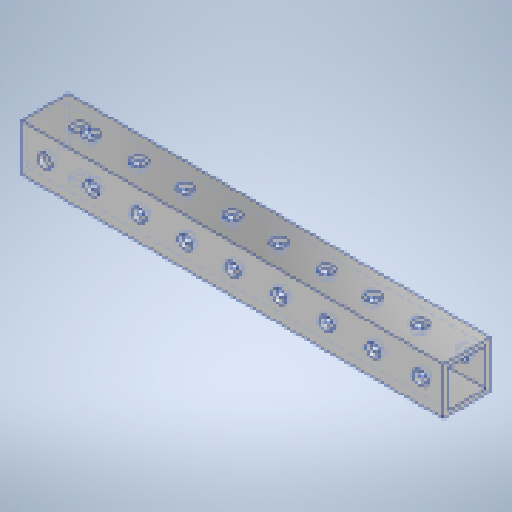
# Autodesk Inventor part: 10x10x60
Saved by Autodesk Inventor 2025 (Build 290162000, 162)
## iProperties
Created: 2025-03-04
Part Number: 10x10x60
Material: アルミニウム 6061
Document SubType Name: Modeling
Designer: Zhopa
Density: 2.7 g/cm^3
Appearance: アルミニウム - フラット
Mass: 8.06397 g
Surface Area: 63.7758 cm^2
Volume: 2.98666 cm^3
Author: Zhopa
Autodesk Inventor part; units mm, degrees
ref_plane "YZ Plane" through (0, 0, 0) normal (1, 0, 0) x (0, 1, 0)
ref_plane "XZ Plane" through (0, 0, 0) normal (0, 1, 0) x (-1, 0, 0)
ref_plane "XY Plane" through (0, 0, 0) normal (0, 0, 1) x (1, 0, 0)
sketch "Sketch1" plane through (0, 0, 0) normal (1, 0, 0) x (0, 1, 0)
  line L0 (-5, -5) -> (5, -5)
  line L1 (5, -5) -> (5, 5)
  line L2 (5, 5) -> (-5, 5)
  line L3 (-5, 5) -> (-5, -5)
  line L4 (-5, -5) -> (5, 5) construction
  line L5 (5, -5) -> (-5, 5) construction
  line L6 (-4, -4) -> (4, -4)
  line L7 (4, -4) -> (4, 4)
  line L8 (4, 4) -> (-4, 4)
  line L9 (-4, 4) -> (-4, -4)
  line L10 (-4, -4) -> (4, 4) construction
  line L11 (4, -4) -> (-4, 4) construction
  point P0 (0, 0)
  dimension "d0" = 10
  dimension "d1" = 10
  dimension "d2" = 8
  dimension "d3" = 8
  constraints: 24 end point, 4 midpoint, 4 parallel, 2 horizontal, 2 perpendicular
  measures "d0" distance of L2.end L1.end
  measures "d1" distance of L1.end L0.end
  measures "d2" distance of L8.end L7.end
  measures "d3" distance of L7.end L6.end
extrude "Extrusion1" add sketch "Sketch1" along normal blind 90
sketch "Sketch2" plane through (0, -5, 5) normal (0, 0, 1) x (1, 0, 0)
  line L0 (90, 10) -> (90, 0) projected
  line L1 (0, 10) -> (0, 0) projected
  line L2 (5, 5) -> (25.8215, 5)
  point P0 (0, 5)
  point P1 (15, 5)
  point P2 (15, 5)
  point P3 (25, 5)
  point P4 (25, 5)
  point P5 (35, 5)
  point P6 (35, 5)
  point P7 (45, 5)
  point P8 (45, 5)
  point P9 (55, 5)
  point P10 (55, 5)
  point P11 (65, 5)
  point P12 (65, 5)
  point P13 (75, 5)
  point P14 (75, 5)
  point P15 (85, 5)
  dimension "d7" = 5
  dimension "d15" = 10
  dimension "d18" = 10
  constraints: 2 end point, 2 horizontal, 14 other
  measures "d7" distance from line of L1 L2.start
  measures "d15" distance of point (15, 5) L2.start
  measures "d18" distance of L2.start point (15, 5)
hole "Hole1" at (5, 0, 5) at (15, 0, 5) at (25, 0, 5) at (35, 0, 5) at (45, 0, 5) at (55, 0, 5) at (65, 0, 5) at (75, 0, 5) at (85, 0, 5) direction (0, 0, -1) diameter 3 depth 80.45
sketch "Sketch3" plane through (0, 5, 5) normal (0, 1, 0) x (1, 0, 0)
  line L0 (0, 10) -> (0, 0) projected
  line L1 (0, 5) -> (10, 5)
  point P0 (20, 5)
  point P1 (20, 5)
  point P2 (30, 5)
  point P3 (30, 5)
  point P4 (40, 5)
  point P5 (40, 5)
  point P6 (50, 5)
  point P7 (50, 5)
  point P8 (60, 5)
  point P9 (60, 5)
  point P10 (70, 5)
  point P11 (70, 5)
  point P12 (80, 5)
  dimension "d23" = 10
  dimension "d24" = 10
  dimension "d27" = 10
  constraints: 2 end point, 2 horizontal, 12 other
  measures "d23" distance from line of L1.end L0
  measures "d24" distance of L1.end point (20, 5)
  measures "d27" distance of L1.end point (20, 5)
hole "Hole2" at (10, 5, 0) at (20, 5, 0) at (30, 5, 0) at (40, 5, 0) at (50, 5, 0) at (60, 5, 0) at (70, 5, 0) at (80, 5, 0) direction (0, -1, 0) diameter 3 depth 80.45
sketch "Sketch4" plane through (0, 5, 5) normal (0, 1, 0) x (1, 0, 0)
  circle A0 centre (10, 5) radius 1.5 projected
  point P0 (0, 5)
  point P1 (7.5, 5)
  dimension "d39" = 2.5
  measures "d39" distance of A0.centre point (7.5, 5)
hole "Hole3" at (7.5, 5, 0) direction (0, -1, 0) diameter 3 depth 80.45
body "Solid1"
